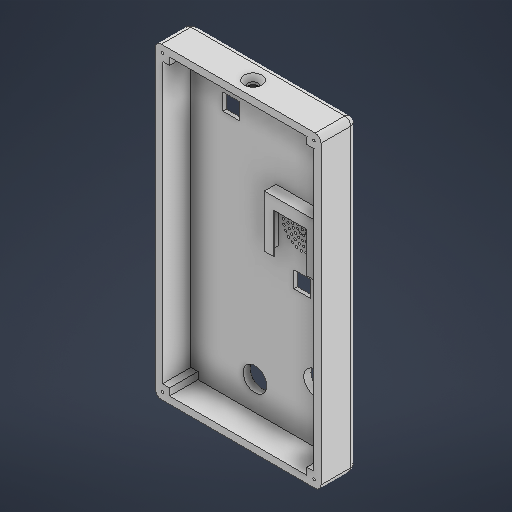
# Autodesk Inventor part: Top_Shell
Saved by Autodesk Inventor 2026.2 (Build 302298010, 298A)
## iProperties
Created: 2026-03-03
Part Number: Top_Shell
Material: Generic
Document SubType Name: Modeling
Designer: kjedr
Density: 1 g/cm^3
Appearance: Default
Author: kjedr
Autodesk Inventor part; units mm, degrees
ref_plane "YZ Plane" through (0, 0, 0) normal (1, 0, 0) x (0, 1, 0)
ref_plane "XZ Plane" through (0, 0, 0) normal (0, 1, 0) x (-1, 0, 0)
ref_plane "XY Plane" through (0, 0, 0) normal (0, 0, 1) x (1, 0, 0)
sketch "Sketch1" plane through (0, 0, 0) normal (0, 0, 1) x (1, 0, 0)
  line L0 (0, 0) -> (88.9, 0)
  line L1 (88.9, 0) -> (88.9, 165.1)
  line L2 (88.9, 165.1) -> (0, 165.1)
  line L3 (0, 165.1) -> (0, 0)
  dimension "d0" = 88.9
  dimension "d1" = 165.1
  constraints: 8 end point, 2 parallel, 1 horizontal, 1 perpendicular
  measures "d0" distance of L2.end L1.end
  measures "d1" distance of L1.end L0.end
extrude "Extrusion1" add sketch "Sketch1" along normal blind 19.05
sketch "Sketch2" plane through (0, 0, 19.05) normal (0, 0, 1) x (1, 0, 0)
  line L0 (3.81, 3.81) -> (85.09, 3.81)
  line L1 (85.09, 3.81) -> (85.09, 161.29)
  line L2 (85.09, 161.29) -> (3.81, 161.29)
  line L3 (3.81, 161.29) -> (3.81, 3.81)
  line L4 (0, 165.1) -> (0, 0) projected
  line L5 (0, 0) -> (88.9, 0) projected
  line L6 (88.9, 0) -> (88.9, 165.1) projected
  line L7 (88.9, 165.1) -> (0, 165.1) projected
  point P0 (88.9, 82.55)
  dimension "d4" = 3.81
  dimension "d5" = 3.81
  dimension "d6" = 3.81
  dimension "d7" = 3.81
  constraints: 8 end point, 2 parallel, 1 horizontal, 1 midpoint, 1 perpendicular
  measures "d4" distance between parallel lines of L4 L3
  measures "d5" distance between parallel lines of L5 L0
  measures "d6" distance from line of point (88.9, 82.55) L1
  measures "d7" distance between parallel lines of L7 L2
extrude "Extrusion2" cut sketch "Sketch2" against normal blind 15.24 contours L3 L2 L1 L0
fillet "Fillet1" radius 3.175 8 edges at (88.9, 165.1, 9.525) (0, 165.1, 9.525) (44.45, 165.1, 0) (88.9, 82.55, 0) (44.45, 0, 0) (0, 82.55, 0) (0, 0, 9.525) (88.9, 0, 9.525)
sketch "Sketch8" plane through (0, 0, 0) normal (0, 0, -1) x (-1, 0, 0)
  circle A0 centre (-63.5, 101.6) radius 12.7 construction
  circle A1 centre (-63.5, 101.6) radius 10.16 construction
  circle A2 centre (-63.5, 101.6) radius 7.62 construction
  circle A3 centre (-63.5, 101.6) radius 5.08 construction
  circle A4 centre (-63.5, 101.6) radius 2.54 construction
  line L0 (-88.9, 161.925) -> (-88.9, 3.175) projected
  line L1 (-85.725, 0) -> (-3.175, 0) projected
  point P0 (0, 0)
  point P1 (-62.6328, 103.9874)
  point P2 (-64.4144, 106.597)
  point P3 (-62.7008, 109.178)
  point P4 (-62.6838, 111.7272)
  point P5 (-65.228, 111.612)
  point P6 (-67.6636, 110.8677)
  point P7 (-69.8376, 109.5411)
  point P8 (-71.6133, 107.7155)
  point P9 (-72.8793, 105.5057)
  point P10 (-73.5559, 103.0504)
  point P11 (-73.6007, 100.5041)
  point P12 (-73.0108, 98.0266)
  point P13 (-71.8234, 95.7736)
  point P14 (-70.1129, 93.8867)
  point P15 (-67.9869, 92.4845)
  point P16 (-65.579, 91.655)
  point P17 (-63.0405, 91.4504)
  point P18 (-60.5308, 91.8835)
  point P19 (-58.2077, 92.9272)
  point P20 (-56.2171, 94.5158)
  point P21 (-54.6842, 96.5496)
  point P22 (-53.7051, 98.9006)
  point P23 (-53.3416, 101.4213)
  point P24 (-53.6163, 103.9532)
  point P25 (-54.512, 106.3373)
  point P26 (-55.9725, 108.4237)
  point P27 (-57.906, 110.0813)
  point P28 (-60.1909, 111.206)
  point P29 (-65.0817, 109.054)
  point P30 (-67.3077, 108.2004)
  point P31 (-69.161, 106.7008)
  point P32 (-70.4601, 104.7018)
  point P33 (-71.078, 102.3992)
  point P34 (-70.954, 100.0183)
  point P35 (-70.1004, 97.7923)
  point P36 (-68.6008, 95.939)
  point P37 (-66.6018, 94.6399)
  point P38 (-64.2992, 94.022)
  point P39 (-61.9183, 94.146)
  point P40 (-59.6923, 94.9996)
  point P41 (-57.839, 96.4992)
  point P42 (-56.5399, 98.4982)
  point P43 (-55.922, 100.8008)
  point P44 (-56.046, 103.1817)
  point P45 (-56.8996, 105.4077)
  point P46 (-58.3992, 107.261)
  point P47 (-60.3982, 108.5601)
  point P48 (-66.3678, 105.7931)
  point P49 (-67.8254, 104.2641)
  point P50 (-68.535, 102.2745)
  point P51 (-68.3741, 100.1682)
  point P52 (-67.3703, 98.3096)
  point P53 (-65.6974, 97.0198)
  point P54 (-63.6445, 96.5221)
  point P55 (-61.5666, 96.9023)
  point P56 (-59.823, 98.0948)
  point P57 (-58.7152, 99.8934)
  point P58 (-58.4348, 101.9871)
  point P59 (-59.0301, 104.0138)
  point P60 (-60.3984, 105.6232)
  point P61 (-62.3029, 106.5369)
  point P62 (-64.575, 103.9013)
  point P63 (-65.8874, 102.4672)
  point P64 (-65.8013, 100.525)
  point P65 (-64.3672, 99.2126)
  point P66 (-62.425, 99.2987)
  point P67 (-61.1126, 100.7328)
  point P68 (-61.1987, 102.675)
  dimension "d39" = 20.32
  dimension "d40" = 15.24
  dimension "d41" = 10.16
  dimension "d42" = 5.08
  dimension "d38" = 25.4
  dimension "d45" = 360
  dimension "d49" = 360
  dimension "d53" = 360
  dimension "d57" = 360
  dimension "d66" = 25.4
  dimension "d67" = 101.6
  constraints: 5 coincident, 1 centre point, 84 other
  measures "d38" diameter of A0
  measures "d66" distance from line of L0 A0.centre
  measures "d67" distance from line of L1 A0.centre
hole "Hole1" at (63.5, 101.6, 0) at (62.6328, 103.9874, 0) at (64.4144, 106.597, 0) at (62.7008, 109.178, 0) at (62.6838, 111.7272, 0) at (65.228, 111.612, 0) at (67.6636, 110.8677, 0) at (69.8376, 109.5411, 0) at (71.6133, 107.7155, 0) at (72.8793, 105.5057, 0) at (73.5559, 103.0504, 0) at (73.6007, 100.5041, 0) at (73.0108, 98.0266, 0) at (71.8234, 95.7736, 0) at (70.1129, 93.8867, 0) at (67.9869, 92.4845, 0) at (65.579, 91.655, 0) at (63.0405, 91.4504, 0) at (60.5308, 91.8835, 0) at (58.2077, 92.9272, 0) at (56.2171, 94.5158, 0) at (54.6842, 96.5496, 0) at (53.7051, 98.9006, 0) at (53.3416, 101.4213, 0) at (53.6163, 103.9532, 0) at (54.512, 106.3373, 0) at (55.9725, 108.4237, 0) at (57.906, 110.0813, 0) at (60.1909, 111.206, 0) at (65.0817, 109.054, 0) at (67.3077, 108.2004, 0) at (69.161, 106.7008, 0) at (70.4601, 104.7018, 0) at (71.078, 102.3992, 0) at (70.954, 100.0183, 0) at (70.1004, 97.7923, 0) at (68.6008, 95.939, 0) at (66.6018, 94.6399, 0) at (64.2992, 94.022, 0) at (61.9183, 94.146, 0) at (59.6923, 94.9996, 0) at (57.839, 96.4992, 0) at (56.5399, 98.4982, 0) at (55.922, 100.8008, 0) at (56.046, 103.1817, 0) at (56.8996, 105.4077, 0) at (58.3992, 107.261, 0) at (60.3982, 108.5601, 0) at (66.3678, 105.7931, 0) at (67.8254, 104.2641, 0) direction (0, 0, 1) diameter 1.27 end through all and at (68.535, 102.2745, 0) (68.3741, 100.1682, 0) (67.3703, 98.3096, 0) (65.6974, 97.0198, 0) (63.6445, 96.5221, 0) (61.5666, 96.9023, 0) (59.823, 98.0948, 0) (58.7152, 99.8934, 0) (58.4348, 101.9871, 0) (59.0301, 104.0138, 0) (60.3984, 105.6232, 0) (62.3029, 106.5369, 0) (64.575, 103.9013, 0) (65.8874, 102.4672, 0) (65.8013, 100.525, 0) (64.3672, 99.2126, 0) (62.425, 99.2987, 0) (61.1126, 100.7328, 0) (61.1987, 102.675, 0)
sketch "Sketch9" plane through (0, 0, 3.81) normal (0, 0, 1) x (1, 0, 0)
  line L0 (49.53, 115.57) -> (77.47, 115.57)
  line L1 (77.47, 115.57) -> (77.47, 87.63)
  line L2 (77.47, 87.63) -> (49.53, 87.63)
  line L3 (49.53, 87.63) -> (49.53, 115.57)
  circle A0 centre (63.5, 101.6) radius 0.635 projected
  line L4 (49.53, 115.57) -> (77.47, 87.63) construction
  line L5 (77.47, 115.57) -> (49.53, 87.63) construction
  point P0 (0, 0)
  dimension "d68" = 27.94
  dimension "d69" = 27.94
  constraints: 12 end point, 2 midpoint, 2 parallel, 1 horizontal, 1 perpendicular
  measures "d68" distance of L1.end L2.end
  measures "d69" distance of L0.end L1.end
sketch "Sketch10" plane through (3.175, 165.1, 19.05) normal (0, 1, 0) x (1, 0, 0)
  line L0 (0, 15.875) -> (82.55, 15.875) projected
  point P0 (-3.175, 19.05)
  point P1 (41.275, 7.9375)
  point P2 (41.275, 15.875)
  constraints: 1 midpoint, 1 vertical alignment
hole "Hole2" at (44.45, 165.1, 11.1125) direction (0, -1, 0) diameter 5.08 depth 3.81 tip angle 118 countersink diameter 9.525 countersink angle 82
sketch "Sketch12" plane through (0, 0, 0) normal (0, 0, -1) x (-1, 0, 0)
  point P0 (0, 0)
sketch "Sketch14" plane through (0, 0, 0) normal (0, 0, -1) x (-1, 0, 0)
  line L0 (-79.719, 90.81) -> (-9.181, 90.81) construction
  line L1 (-9.181, 90.81) -> (-9.181, 6.81) construction
  line L2 (-9.181, 6.81) -> (-79.719, 6.81) construction
  line L3 (-79.719, 6.81) -> (-79.719, 90.81) construction
  circle A0 centre (-75.2472, 83.516) radius 1.6
  circle A1 centre (-13.6268, 83.516) radius 1.6
  circle A2 centre (-75.2472, 22.81) radius 1.6
  circle A3 centre (-13.6268, 22.81) radius 1.6
  line L4 (-85.725, 161.925) -> (-3.175, 161.925) projected
  line L5 (-85.09, 3.81) -> (-3.81, 3.81) projected
  point P0 (0, 0)
  point P1 (-44.45, 90.81)
  point P2 (-44.45, 125.7733)
  point P3 (-70.739, 33.81)
  point P4 (-38.181, 19.31)
  point P5 (-44.45, 6.81)
  point P6 (-44.45, 161.925)
  dimension "d88" = 70.538
  dimension "d89" = 84
  dimension "d90" = 3.2
  dimension "d91" = 60.706
  dimension "d92" = 61.6204
  dimension "d93" = 16
  dimension "d94" = 4.4458
  dimension "d96" = 27
  dimension "d97" = 8.98
  dimension "d98" = 12.5
  dimension "d99" = 29
  dimension "d101" = 3
  constraints: 8 end point, 4 centre point, 4 vertical alignment, 3 equal radius, 3 midpoint, 2 horizontal alignment, 2 parallel, 1 horizontal, 1 perpendicular
  measures "d88" distance of L1.end L2.end
  measures "d89" distance of L0.end L1.end
  measures "d90" diameter of A0
  measures "d91" distance of A2.centre A0.centre
  measures "d92" distance of A3.centre A2.centre
  measures "d93" distance from line of L2 A3.centre
  measures "d94" distance from line of L1 A3.centre
  measures "d96" distance from line of L2 point (-70.739, 33.81)
  measures "d97" distance from line of L3 point (-70.739, 33.81)
  measures "d98" distance from line of L2 point (-38.181, 19.31)
  measures "d99" distance from line of L1 point (-38.181, 19.31)
  measures "d101" distance between parallel lines of L5 L2
hole "Hole4" at (70.739, 33.81, 0) at (38.181, 19.31, 0) direction (0, 0, 1) diameter 12.7 end through all
extrude "Extrusion6" add sketch "Sketch9" along normal blind 6.35 contours L0 L1 L2 L3 | A0
sketch "Sketch16" plane through (49.53, 87.63, 3.81) normal (0, -1, 0) x (1, 0, 0)
  line L0 (26.67, 0) -> (1.27, 0)
  line L1 (1.27, 0) -> (1.27, 5.715)
  line L2 (1.27, 5.715) -> (26.67, 5.715)
  line L3 (26.67, 5.715) -> (26.67, 0)
  line L4 (27.94, 0) -> (0, 0) projected
  line L5 (0, 6.35) -> (27.94, 6.35) projected
  line L6 (0, 0) -> (0, 6.35) projected
  line L7 (22.86, 5.715) -> (5.08, 5.715)
  line L8 (5.08, 5.715) -> (5.08, 6.35)
  line L9 (5.08, 6.35) -> (22.86, 6.35)
  line L10 (22.86, 6.35) -> (22.86, 5.715)
  point P0 (-49.53, -3.81)
  point P1 (22.86, 6.35)
  point P2 (5.08, 5.715)
  dimension "d111" = 0
  dimension "d112" = 25.4
  dimension "d113" = 0.635
  dimension "d114" = 1.27
  dimension "d115" = 3.81
  dimension "d121" = 3.81
  constraints: 16 end point, 4 parallel, 2 horizontal, 2 perpendicular, 2 point on line
  measures "d111" distance between parallel lines of L4 L0
  measures "d112" distance between parallel lines of L3 L1
  measures "d113" distance between parallel lines of L5 L2
  measures "d114" distance between parallel lines of L6 L1
  measures "d115" distance between parallel lines of L3 L10
  measures "d121" distance between parallel lines of L1 L8
extrude "Extrusion7" cut sketch "Sketch16" against normal blind 26.67 contours L0 L1 L2 L3
extrude "Extrusion8" cut sketch "Sketch16" against normal blind 21.59 contours L2 L8 L5 L10
sketch "Sketch19" plane through (0, 0, 3.81) normal (0, 0, 1) x (1, 0, 0)
  line L0 (3.81, 161.29) -> (85.09, 161.29) projected
  line L1 (3.81, 161.29) -> (7.62, 161.29)
  line L2 (7.62, 161.29) -> (7.62, 157.48)
  line L3 (7.62, 157.48) -> (3.81, 157.48)
  line L4 (3.81, 157.48) -> (3.81, 161.29)
  line L5 (85.09, 161.29) -> (81.28, 161.29)
  line L6 (81.28, 161.29) -> (81.28, 157.48)
  line L7 (81.28, 157.48) -> (85.09, 157.48)
  line L8 (85.09, 157.48) -> (85.09, 161.29)
  line L9 (85.09, 3.81) -> (3.81, 3.81) projected
  line L10 (3.81, 3.81) -> (7.62, 3.81)
  line L11 (7.62, 3.81) -> (7.62, 7.62)
  line L12 (7.62, 7.62) -> (3.81, 7.62)
  line L13 (3.81, 7.62) -> (3.81, 3.81)
  line L14 (85.09, 3.81) -> (81.28, 3.81)
  line L15 (81.28, 3.81) -> (81.28, 7.62)
  line L16 (81.28, 7.62) -> (85.09, 7.62)
  line L17 (85.09, 7.62) -> (85.09, 3.81)
  point P0 (0, 0)
  dimension "d122" = 3.81
  dimension "d123" = 3.81
  dimension "d124" = 3.81
  dimension "d125" = 3.81
  dimension "d126" = 3.81
  dimension "d127" = 3.81
  dimension "d128" = 3.81
  dimension "d129" = 3.81
  constraints: 32 end point, 8 parallel, 4 horizontal, 4 perpendicular
  measures "d122" distance of L2.end L3.end
  measures "d123" distance of L1.end L2.end
  measures "d124" distance of L7.end L6.end
  measures "d125" distance of L6.end L5.end
  measures "d126" distance of L12.end L11.end
  measures "d127" distance of L11.end L10.end
  measures "d128" distance of L15.end L16.end
  measures "d129" distance of L14.end L15.end
extrude "Extrusion9" add sketch "Sketch19" along normal up to surface (15.24 mm away)
sketch "Sketch20" plane through (0, 0, 19.05) normal (0, 0, 1) x (1, 0, 0)
  line L0 (3.81, 7.62) -> (3.81, 157.48) projected
  line L1 (81.28, 3.81) -> (7.62, 3.81) projected
  line L2 (85.09, 157.48) -> (85.09, 7.62) projected
  line L3 (7.62, 161.29) -> (81.28, 161.29) projected
  point P0 (0, 0)
  point P1 (3.81, 3.81)
  point P2 (85.09, 3.81)
  point P3 (85.09, 161.29)
  point P4 (3.81, 161.29)
  dimension "d132" = 0
  dimension "d133" = 0
  dimension "d134" = 0
  dimension "d135" = 0
  constraints: 2 horizontal alignment, 2 vertical alignment
  measures "d132" distance from line of L0 point (3.81, 3.81)
  measures "d133" distance from line of point (3.81, 3.81) L1
  measures "d134" distance from line of point (85.09, 3.81) L2
  measures "d135" distance from line of point (85.09, 161.29) L3
hole "Hole5" at (3.81, 161.29, 19.05) at (85.09, 161.29, 19.05) at (85.09, 3.81, 19.05) at (3.81, 3.81, 19.05) direction (0, 0, -1) diameter 1.27 depth 15.24
sketch "Sketch21" plane through (0, 0, 0) normal (0, 0, -1) x (-1, 0, 0)
  line L0 (-69.85, 82.55) -> (-57.15, 82.55)
  line L1 (-57.15, 82.55) -> (-57.15, 69.85)
  line L2 (-57.15, 69.85) -> (-69.85, 69.85)
  line L3 (-69.85, 69.85) -> (-69.85, 82.55)
  line L4 (-69.85, 82.55) -> (-57.15, 69.85) construction
  line L5 (-57.15, 82.55) -> (-69.85, 69.85) construction
  line L6 (-31.75, 146.05) -> (-19.05, 146.05)
  line L7 (-19.05, 146.05) -> (-19.05, 133.35)
  line L8 (-19.05, 133.35) -> (-31.75, 133.35)
  line L9 (-31.75, 133.35) -> (-31.75, 146.05)
  line L10 (-31.75, 146.05) -> (-19.05, 133.35) construction
  line L11 (-19.05, 146.05) -> (-31.75, 133.35) construction
  line L12 (-67.945, 80.645) -> (-59.055, 80.645)
  line L13 (-59.055, 80.645) -> (-59.055, 71.755)
  line L14 (-59.055, 71.755) -> (-67.945, 71.755)
  line L15 (-67.945, 71.755) -> (-67.945, 80.645)
  line L16 (-67.945, 80.645) -> (-59.055, 71.755) construction
  line L17 (-59.055, 80.645) -> (-67.945, 71.755) construction
  line L18 (-85.725, 0) -> (-3.175, 0) projected
  circle A0 centre (-63.5, 101.6) radius 0.635 projected
  line L19 (-29.845, 144.145) -> (-20.955, 144.145)
  line L20 (-20.955, 144.145) -> (-20.955, 135.255)
  line L21 (-20.955, 135.255) -> (-29.845, 135.255)
  line L22 (-29.845, 135.255) -> (-29.845, 144.145)
  line L23 (-29.845, 144.145) -> (-20.955, 135.255) construction
  line L24 (-20.955, 144.145) -> (-29.845, 135.255) construction
  line L25 (0, 3.175) -> (0, 161.925) projected
  line L26 (-3.175, 165.1) -> (-85.725, 165.1) projected
  point P0 (0, 0)
  point P1 (-63.5, 76.2)
  point P2 (-25.4, 139.7)
  dimension "d143" = 12.7
  dimension "d144" = 12.7
  dimension "d145" = 12.7
  dimension "d146" = 12.7
  dimension "d147" = 8.89
  dimension "d148" = 76.2
  dimension "d149" = 25.4
  dimension "d150" = 8.89
  dimension "d151" = 8.89
  dimension "d152" = 25.4
  dimension "d153" = 25.4
  constraints: 48 end point, 8 midpoint, 8 parallel, 4 horizontal, 4 perpendicular, 1 point on line
  measures "d143" distance of L1.end L2.end
  measures "d144" distance of L0.end L1.end
  measures "d145" distance of L7.end L8.end
  measures "d146" distance of L6.end L7.end
  measures "d147" distance of L13.end L14.end
  measures "d148" distance from line of L18 point (-63.5, 76.2)
  measures "d149" distance of A0.centre point (-63.5, 76.2)
  measures "d150" distance of L20.end L21.end
  measures "d151" distance of L19.end L20.end
  measures "d152" distance from line of L25 point (-25.4, 139.7)
  measures "d153" distance from line of point (-25.4, 139.7) L26
extrude "Extrusion10" cut sketch "Sketch21" against normal blind 3.81 contours L12 L13 L14 L15 | L19 L20 L21 L22
extrude "Extrusion11" cut sketch "Sketch21" against normal blind 1.905 contours L0 L1 L2 L3 | L6 L7 L8 L9 | L19 L20 L21 L22
body "Solid1"
